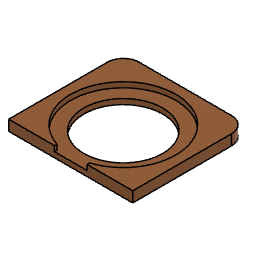
electrode puck v2 insulation v8 (Autodesk Fusion 360 design; units mm, degrees)
Autodesk Fusion 360 part; units mm, degrees
sketch "Sketch1" plane through (0, 0, 0) normal (0, 1, 0) x (1, 0, 0)
  line L0 (0, 0) -> (12, 0)
  line L1 (12, 0) -> (12, -11)
  line L2 (12, -11) -> (0, -11)
  line L3 (0, -11) -> (0, 0)
  circle A0 centre (6, -6) radius 3.75
  line L4 (6, -11) -> (6, -6) construction
  line L5 (1, -11) -> (1, -1)
  line L6 (1, -1) -> (11, -1)
  line L7 (11, -1) -> (11, -11)
  circle A1 centre (6, -6) radius 5
  line L8 (4.45, -10.7537) -> (4.45, -11)
  line L9 (7.55, -10.7537) -> (7.55, -11)
  arc A2 (3.299, -11) -> (0.701, -11) centre (2, -11.75) ccw
  dimension "d1" = 12
  dimension "d2" = 11
  dimension "d3" = 5
  dimension "d4" = 7.5
  dimension "d5" = 1
  dimension "d11" = 10
  dimension "d12" = 3.1
  dimension "d14" = 1.5
  dimension "d15" = 4
  dimension "d16" = 0.75
  constraint horizontal L0
  constraint vertical L1
  constraint horizontal L2
  constraint vertical L3
  constraint coincident L0.start L3.end
  constraint midpoint L2 L4.start
  constraint coincident A0.centre L4.end
  constraint perpendicular L2 L4
  constraint concentric A0 A1
  constraint coincident A1 L8.start
  constraint coincident L2 L8.end
  constraint perpendicular L2 L8
  constraint coincident A1 L9.start
  constraint coincident L2 L9.end
  constraint perpendicular L2 L9
  constraint symmetric L4 L8 L9
  constraint coincident L2 A2.start
  constraint coincident L2 A2.end
  measures "d1" distance of L1.end L2.end
  measures "d2" distance of L0.end L1.end
  measures "d3" distance of L2 A0.centre
  measures "d4" diameter of A0
  measures "d11" diameter of A1
  measures "d12" distance of L8 L9
  measures "d14" radius of A2
  measures "d15" distance of L4 A2.centre
  measures "d16" distance of L2 A2.centre
extrude "Extrude1" add sketch "Sketch1" along normal blind 1 contours L0 L1 L2 L3 L5 L6 L7 A2 | L2 L5 A2 | L2 L7 A1 L9 | L2 L5 A2 | L2 L5 A1 L8 A2 | L6 L7 A1 | L5 L6 A1
extrude "Extrude2" add sketch "Sketch1" along normal blind 0.5 contours L2 L7 A1 L9 | L2 L5 A2 | L2 L5 A1 L8 A2 | L2 A1 L9 | L6 L7 A1 | A1 | L5 L6 A1 | L2 A1 L8 picked at (2.4911, -10.9389)
fillet "Fillet1" radius 1.5 2 edges at (12, 0.5, 0) (0, 0.5, 0)
move_face "OffsetFaces1" offset -0.1 3 faces at (12, 0.3333, 4.6667) (4.5, 0.3333, 0) (0, 0.3333, 7.8333)
